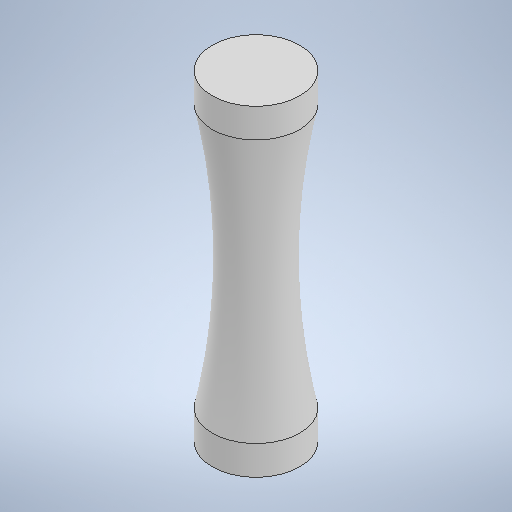
# Autodesk Inventor part: Supporter
Saved by Autodesk Inventor 2025.1 (Build 291241020, 241B)
## iProperties
Created: 2024-09-21
Part Number: Supporter
Material: 일반
Document SubType Name: Modeling
Designer: daare
Density: 1 g/cm^3
Appearance: 기본값
Author: daare
Autodesk Inventor part; units mm, degrees
ref_plane "YZ Plane" through (0, 0, 0) normal (1, 0, 0) x (0, 1, 0)
ref_plane "XZ Plane" through (0, 0, 0) normal (0, 1, 0) x (-1, 0, 0)
ref_plane "XY Plane" through (0, 0, 0) normal (0, 0, 1) x (1, 0, 0)
sketch "스케치1" plane through (0, 0, 0) normal (0, 0, 1) x (1, 0, 0)
  line L0 (-7.5, -2.5) -> (7.5, -2.5)
  line L1 (7.5, -2.5) -> (7.5, 2.5)
  line L2 (7.5, 2.5) -> (-7.5, 2.5)
  line L3 (-7.5, 2.5) -> (-7.5, -2.5)
  line L4 (-7.5, -2.5) -> (7.5, 2.5) construction
  line L5 (7.5, -2.5) -> (-7.5, 2.5) construction
  line L6 (-7.5, 2.5) -> (7.5, 2.5)
  line L7 (7.5, 2.5) -> (7.5, 52.5)
  line L8 (7.5, 52.5) -> (-7.5, 52.5)
  line L9 (-7.5, 52.5) -> (-7.5, 2.5)
  arc A0 (-7.5, 2.5) -> (-7.5, 47.5) centre (-115.1743, 25) ccw
  line L10 (0, 52.5) -> (0, -2.5)
  point P0 (0, 0)
  dimension "d0" = 15
  dimension "d1" = 5
  dimension "d2" = 55
  dimension "d3" = 5
  dimension "d4" = 110
  constraints: 22 end point, 4 midpoint, 4 parallel, 2 horizontal, 2 perpendicular, 2 point on circle, 1 centre point, 1 point on line
  measures "d0" distance of L1.end L2.end
  measures "d1" distance of L0.end L1.end
  measures "d2" distance between parallel lines of L0 L8
  measures "d3" distance from line of L8 A0.end
  measures "d4" radius of A0
revolve "회전1" add sketch "스케치1" angle 360 about axis through (0, 52.5, 0) along (0, -1, 0) contours L3 L2 L10 L0 | A0 L9 L8 L10 L2
